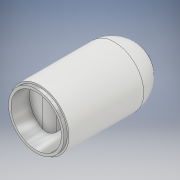
# Autodesk Inventor part: Pencil Cab
Saved by Autodesk Inventor 2018 (Build 220112000, 112)
## iProperties
Created: 2020-01-09
Part Number: Pencil Cab
Material: Generic
Document SubType Name: Modeling
Designer: AOFUser
Density: 1 g/cm^3
Appearance: Default
Author: AOFUser
Autodesk Inventor part; units mm, degrees
ref_plane "YZ Plane" through (0, 0, 0) normal (1, 0, 0) x (0, 1, 0)
ref_plane "XZ Plane" through (0, 0, 0) normal (0, 1, 0) x (-1, 0, 0)
ref_plane "XY Plane" through (0, 0, 0) normal (0, 0, 1) x (1, 0, 0)
sketch "Sketch1" plane through (0, 0, 0) normal (0, 1, 0) x (-1, 0, 0)
  line L0 (0, 0) -> (0, -16.256)
  line L1 (0, -16.256) -> (0, -11.811)
  arc A0 (0, -16.256) -> (4.445, -11.811) centre (-0.6095, -11.2015) ccw
  line L2 (0, -16.256) -> (0, -15.3712)
  line L3 (0, -15.3712) -> (0, -14.8015)
  line L4 (4.445, -11.811) -> (4.445, -8.128)
  line L5 (0, 0) -> (0, -2.794)
  line L6 (0, -2.794) -> (4.445, -2.794)
  line L7 (4.445, -2.794) -> (4.445, -8.128)
  line L8 (0, 0) -> (0, -0.508)
  line L9 (4.445, -0.508) -> (4.445, -2.794)
  line L10 (4.445, -0.508) -> (4.191, -0.508)
  line L11 (4.191, -0.508) -> (4.191, 0)
  line L12 (4.191, 0) -> (3.81, 0)
  line L13 (3.81, 0) -> (3.81, -2.794)
  line L14 (4.191, -0.508) -> (4.191, -2.794)
  line L15 (2.0957, -15.5144) -> (2.0957, -11.7468)
  line L16 (2.681, -15.0863) -> (2.681, -11.7468)
  line L17 (2.681, -11.7468) -> (2.0957, -11.7468)
  dimension "d0" = 16.256
  dimension "d2" = 4.445
  dimension "d3" = 2.794
  dimension "d4" = 0.508
  dimension "d5" = 0.254
  dimension "d7" = 0.381
  constraints: 36 end point, 8 point on line, 4 perpendicular, 4 point on circle, 3 vertical, 1 centre point, 1 horizontal
  measures "d0" distance of L0.start L0.end
  measures "d2" distance of L0.end L1.end
  measures "d3" distance of L0.start L5.end
  measures "d4" distance of L0.start L8.end
  measures "d5" distance of L9.start L10.end
  measures "d7" distance of L11.end L12.end
revolve "Revolution1" add sketch "Sketch1" angle 360 about axis through (0, 0, 0) along (0, 0, -1) contours L6 L7 L4 A0 L16 L17 L15 L0 | L13 L12 L11 L14 L6 | L14 L10 L9 L6
sketch "Sketch2" plane through (0, 0, -2.794) normal (0, 0, 1) x (1, 0, 0)
  line L0 (0, 0) -> (0.762, 0)
  line L1 (0.762, 0) -> (0.762, 3.733)
  circle A0 centre (0, 0) radius 3.81 projected
  line L2 (0.762, 0) -> (0.762, -3.733)
  line L3 (0, 0) -> (-0.762, 0)
  line L4 (-0.762, 0) -> (-0.762, 3.733)
  line L5 (-0.762, 0) -> (-0.762, -3.733)
  dimension "d9" = 0.762
  dimension "d10" = 0.762
  constraints: 12 end point, 4 point on circle, 2 horizontal, 2 perpendicular, 1 vertical
  measures "d9" distance of L0.start L0.end
  measures "d10" distance of L3.start L3.end
extrude "Extrusion1" cut sketch "Sketch2" against normal blind 8.89 contours L3 L4 A0 L1 L0 | L0 L2 A0 L5 L3
fillet "Fillet1" radius 1.016 6 edges at (-0.762, -1.8665, -2.794) (-0.762, 1.8665, -2.794) (0.762, 1.8665, -2.794) (0.762, -1.8665, -2.794) (0, 3.81, -11.684) (0, -3.81, -11.684)
body "Solid1"
